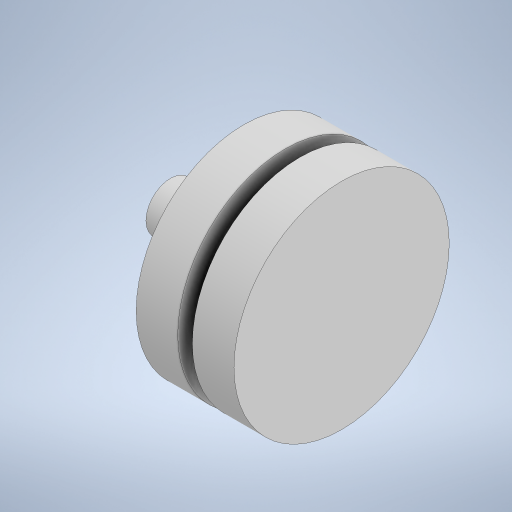
# Autodesk Inventor part: head and tail wheel
Saved by Autodesk Inventor 2024 (Build 280153000, 153)
## iProperties
Created: 2023-06-19
Part Number: head and tail wheel
Material: Generic
Document SubType Name: Modeling
Designer: dipes
Density: 1 g/cm^3
Appearance: Default
Author: dipes
Autodesk Inventor part; units mm, degrees
ref_plane "YZ Plane" through (0, 0, 0) normal (1, 0, 0) x (0, 1, 0)
ref_plane "XZ Plane" through (0, 0, 0) normal (0, 1, 0) x (-1, 0, 0)
ref_plane "XY Plane" through (0, 0, 0) normal (0, 0, 1) x (1, 0, 0)
sketch "Sketch1" plane through (0, 0, 0) normal (1, 0, 0) x (0, 1, 0)
  circle A0 centre (0, 0) radius 18
  dimension "d0" = 36
  constraints: 1 centre point, 1 coincident
  measures "d0" diameter of A0
extrude "Extrusion1" add sketch "Sketch1" along normal blind 10 and the other way blind 10
sketch "Sketch2" plane through (10, 0, 0) normal (1, 0, 0) x (0, 0, -1)
  circle A0 centre (0, 0) radius 22
  dimension "d5" = 44
  constraints: 1 centre point, 1 coincident
  measures "d5" diameter of A0
extrude "Extrusion2" add sketch "Sketch2" against normal blind 8.5
sketch "Sketch3" plane through (-10, 0, 0) normal (-1, 0, 0) x (0, 0, 1)
  circle A0 centre (0, 0) radius 22
  dimension "d8" = 44
  constraints: 1 centre point, 1 coincident
  measures "d8" diameter of A0
extrude "Extrusion3" add sketch "Sketch3" against normal blind 8.5
sketch "Sketch4" plane through (-10, 0, 0) normal (-1, 0, 0) x (0, 0, 1)
  circle A0 centre (0, 0) radius 2.5
  dimension "d11" = 5
  constraints: 1 centre point, 1 coincident
  measures "d11" diameter of A0
extrude "Extrusion4" add sketch "Sketch4" along normal blind 15
sketch "Sketch5" plane through (-10, 0, 0) normal (-1, 0, 0) x (0, 0, 1)
  circle A0 centre (0, 0) radius 2.5 projected
  circle A1 centre (0, 0) radius 5
  dimension "d14" = 10
  constraints: 1 centre point, 1 coincident
  measures "d14" diameter of A1
sketch "Sketch7" plane through (-25, 0, 0) normal (-1, 0, 0) x (0, 0, 1)
  point P0 (0, 0)
extrude "Extrusion6" add sketch "Sketch5" along normal blind 15 contours A0 | A1
sketch "Sketch8" plane through (10, 0, 0) normal (1, 0, 0) x (0, 0, -1)
  point P0 (0, 0)
  point P1 (0, 0)
  dimension "d20" = 0
  constraints: 1 coincident, 2 other
extrude "Extrusion7" [suppressed]
sketch "Sketch10" plane through (-25, 0, 0) normal (-1, 0, 0) x (0, 0, 1)
  line L0 (1.75, -2.6) -> (1.75, 2.6) projected
  line L1 (-1.75, -2.6) -> (1.75, -2.6)
  line L2 (1.75, -2.6) -> (1.75, 2.6)
  line L3 (1.75, 2.6) -> (-1.75, 2.6)
  line L4 (-1.75, 2.6) -> (-1.75, -2.6)
  line L5 (-1.75, -2.6) -> (1.75, 2.6) construction
  line L6 (1.75, -2.6) -> (-1.75, 2.6) construction
  point P0 (0, 0)
  dimension "d27" = 3.5
  constraints: 12 end point, 2 midpoint, 2 parallel, 1 horizontal, 1 perpendicular
  measures "d27" distance of L3.end L0.end
extrude "Extrusion9" cut sketch "Sketch10" against normal blind 10
sketch "Sketch13" plane through (-15, 0, 0) normal (-1, 0, 0) x (0, 0, 1)
  circle A0 centre (0, 0) radius 0.11 projected
  circle A1 centre (0, 0) radius 0.11
  dimension "d33" = 0.22
  constraints: 1 centre point, 1 coincident
  measures "d33" diameter of A1
extrude "Extrusion11" cut sketch "Sketch13" against normal blind 10
body "Solid1"
